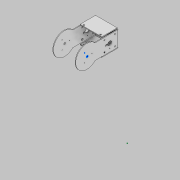
# Autodesk Inventor part: wzmocnienie2M1Dedit
Saved by Autodesk Inventor 2021 (Build 250183000, 183)
## iProperties
Created: 2021-09-03
Part Number: wzmocnienie2M1Dedit
Material: Ogólny
Document SubType Name: Konstrukcja blachowa
Designer: marci
Density: 1 g/cm^3
Sheet Metal Rule: Domyślny_mm
Appearance: Domyślna
Author: marci
Autodesk Inventor part; units mm, degrees
ref_plane "YZ Plane" through (0, 0, 0) normal (1, 0, 0) x (0, 1, 0)
sketch "Szkic1" plane through (0, 0, 0) normal (1, 0, 0) x (0, 1, 0)
  circle A0 centre (425.9063, 179.6758) radius 4.1
  line L0 (460.0949, 39.6758) -> (391.7177, 39.6758)
  line L1 (428.4063, 86.5216) -> (428.4063, 97.3591)
  line L2 (428.4063, 97.3591) -> (423.4063, 97.3591)
  line L3 (423.4063, 97.3591) -> (423.4063, 86.5216)
  arc A1 (423.4063, 86.5216) -> (428.4063, 86.5216) centre (425.9063, 77.8758) ccw
  circle A2 centre (406.1366, 78.0058) radius 1.65
  line L4 (460.0949, 143.191) -> (460.0949, 39.6758)
  arc A3 (460.0949, 143.191) -> (391.7177, 143.191) centre (425.9063, 179.6758) ccw
  line L5 (391.7177, 39.6758) -> (391.7177, 143.191)
  circle A4 centre (449.4563, 101.4258) radius 2.6
  circle A5 centre (402.3563, 101.4258) radius 2.6
  circle A6 centre (402.3563, 54.3258) radius 2.6
  circle A7 centre (449.4563, 54.3258) radius 2.6
  line L6 (423.4063, 95.8758) -> (428.4063, 95.8758)
  point P0 (0, 0)
  point P1 (391.7177, 143.191)
  dimension "d0" = 5.2
  dimension "d1" = 50
  dimension "d2" = 8.2
  dimension "d3" = 9
  dimension "d4" = 3.3
  dimension "d5" = 31.6886
  dimension "d6" = 36.6886
  dimension "d7" = 68.3772
  dimension "d8" = 1.4833
  dimension "d9" = 57.6833
  dimension "d10" = 0
  dimension "d11" = 45.8319
  dimension "d12" = 45.8319
  dimension "d13" = 57.6833
  dimension "d14" = 0
  dimension "d15" = 10.6386
  dimension "d16" = 4.0667
  dimension "d17" = 10.6386
  dimension "d18" = 43.0333
  dimension "d19" = 31.6886
  dimension "d20" = 0
  dimension "d21" = 31.6886
  dimension "d22" = 10.8375
  dimension "d23" = 31.6886
  dimension "d24" = 10.8375
  dimension "d25" = 34.1886
  dimension "d26" = 34.1886
  dimension "d27" = 36.6886
  dimension "d28" = 0
  dimension "d29" = 36.6886
  dimension "d30" = 10.8375
  dimension "d31" = 36.6886
  dimension "d32" = 22.2697
  dimension "d33" = 19.3533
  dimension "d34" = 57.7386
  dimension "d35" = 4.0667
  dimension "d36" = 57.7386
  dimension "d37" = 43.0333
  dimension "d38" = 68.3772
  dimension "d39" = 45.8319
  dimension "d40" = 68.3772
  dimension "d41" = 57.6833
  constraints: 14 end point, 8 centre point, 4 point on circle, 3 equal radius, 3 parallel, 3 perpendicular, 1 concentric
  measures "d0" diameter of A4
  measures "d1" radius of A3
  measures "d2" diameter of A0
  measures "d3" radius of A1
  measures "d4" diameter of A2
  measures "d5" distance between parallel lines of L4 L1
  measures "d6" distance between parallel lines of L4 L3
  measures "d7" distance between parallel lines of L4 L5
  measures "d8" distance between parallel lines of L6 L2
  measures "d9" distance between parallel lines of L2 L0
  measures "d10" distance from line of A3.start L4
  measures "d11" distance from line of A3.start L2
  measures "d12" distance from line of L4.start L2
  measures "d13" distance from line of L4.end L2
  measures "d14" distance from line of L0.start L4
  measures "d15" distance from line of A4.centre L4
  measures "d16" distance from line of A4.centre L2
  measures "d17" distance from line of A7.centre L4
  measures "d18" distance from line of A7.centre L2
  measures "d19" distance from line of L2.start L4
  measures "d20" distance from line of L1.end L2
  measures "d21" distance from line of L6.end L4
  measures "d22" distance from line of L1.start L2
  measures "d23" distance from line of A1.end L4
  measures "d24" distance from line of A1.end L2
  measures "d25" distance from line of A0.centre L4
  measures "d26" distance from line of A1.centre L4
  measures "d27" distance from line of L2.end L4
  measures "d28" distance from line of L3.start L2
  measures "d29" distance from line of L6.start L4
  measures "d30" distance from line of L3.end L2
  measures "d31" distance from line of A1.start L4
  measures "d32" distance from line of A2.centre L1
  measures "d33" distance from line of A2.centre L2
  measures "d34" distance from line of A5.centre L4
  measures "d35" distance from line of A5.centre L2
  measures "d36" distance from line of A6.centre L4
  measures "d37" distance from line of A6.centre L2
  measures "d38" distance from line of A3.end L4
  measures "d39" distance from line of L5.end L2
  measures "d40" distance from line of L0.end L4
  measures "d41" distance from line of L5.start L2
extrude "Wyciągnięcie proste1" add sketch "Szkic1" along normal blind 102.5
ref_plane "Płaszczyzna konstrukcyjna1" through (102.5, 425.9063, 229.6758) normal (0, 0, -1) x (-1, 0, 0)
sketch "Szkic2" plane through (102.5, 425.9063, 229.6758) normal (0, 0, -1) x (-1, 0, 0)
  line L0 (102.5, 50) -> (0, 50) projected
  line L1 (99.5, 50) -> (99.5, -50)
  line L2 (102.5, -50) -> (0, -50) projected
  line L3 (3, 50) -> (3, -50)
  line L4 (102.5, 50) -> (102.5, -50) projected
  line L5 (0, 50) -> (0, -50) projected
  line L6 (99.5, 50) -> (3, 50)
  line L7 (3, -50) -> (99.5, -50)
  point P0 (102.5, -425.9063)
  point P1 (102.5, 34.1886)
  point P2 (102.5, -34.1886)
  point P3 (0, 34.1886)
  point P4 (0, -34.1886)
  point P5 (3, 50)
  dimension "d44" = 3
  dimension "d45" = 3
  constraints: 8 end point, 2 point on line, 2 vertical, 1 collinear, 1 horizontal
  measures "d44" distance between parallel lines of L4 L1
  measures "d45" distance between parallel lines of L5 L3
extrude "Wyciągnięcie proste2" cut sketch "Szkic2" along normal blind 187 contours L1 L2 L3 L0
fillet "Zaokrąglenie1" radius 2 2 edges at (0, 425.9063, 39.6758) (102.5, 425.9063, 39.6758)
sketch "Szkic3" plane through (102.5, 0, 0) normal (1, 0, 0) x (0, 0, -1)
  circle A0 centre (-179.6758, 425.9063) radius 4.1 projected
  circle A1 centre (-179.6758, 425.9063) radius 50
  line L0 (-143.0152, 391.9063) -> (-39.6758, 391.9063)
  line L1 (-39.6758, 391.7177) -> (-39.6758, 460.0949) projected
  line L2 (-143.0152, 459.9063) -> (-39.6758, 459.9063)
  line L3 (-39.6758, 425.9063) -> (-57.2336, 425.9063)
  line L4 (-143.191, 391.7177) -> (-41.6758, 391.7177) projected
  line L5 (-41.6758, 460.0949) -> (-143.191, 460.0949) projected
  line L6 (-39.6758, 391.7177) -> (-41.6758, 391.7177) projected
  line L7 (-41.6758, 460.0949) -> (-39.6758, 460.0949) projected
  point P0 (0, 0)
  dimension "d49" = 68
  dimension "d50" = 34
  dimension "d51" = 100
  constraints: 6 end point, 2 horizontal, 2 point on circle, 2 point on line, 1 centre point, 1 coincident, 1 midpoint, 1 parallel
  measures "d49" distance between parallel lines of L2 L0
  measures "d50" distance between parallel lines of L3 L0
  measures "d51" diameter of A1
extrude "Wyciągnięcie proste3" cut sketch "Szkic3" against normal through all contours A1 L5 L7 L1 L2 | L0 L1 L6 L4 A1
sketch "Szkic4" plane through (102.5, 459.9063, 143.0152) normal (0, 1, 0) x (1, 0, 0)
  line L0 (-3, 100.3394) -> (-99.5, 100.3394) projected
  line L1 (-100.5, 103.3394) -> (-2, 103.3394) projected
  line L2 (-3, 100.3394) -> (-3, 103.3394)
  line L3 (-2, 103.3394) -> (-100.5, 103.3394) projected
  line L4 (0, 101.3394) -> (0, 0) projected
  line L5 (-99.5, 100.3394) -> (-99.5, 103.3394)
  point P0 (-102.5, 143.0152)
  point P1 (-3, 103.3394)
  dimension "d54" = 3
  constraints: 4 end point, 3 point on line, 2 perpendicular
  measures "d54" distance between parallel lines of L4 L2
extrude "Wyciągnięcie proste4" add sketch "Szkic4" along normal blind 3
ref_plane "Płaszczyzna konstrukcyjna2" through (102.5, 425.9063, 41.6758) normal (0, -1, 0) x (1, 0, 0)
mirror "Odbij1" about plane through (102.5, 425.9063, 41.6758) normal (0, -1, 0) of "Wyciągnięcie proste4"
sketch "Szkic5" plane through (2, 391.9063, 39.6758) normal (0, 0, -1) x (-1, 0, 0)
  line L0 (-1, 71) -> (-97.5, 71) projected
  line L1 (-97.5, 71) -> (-97.5, 74)
  line L2 (-97.5, -16) -> (-97.5, 84) projected
  line L3 (-97.5, 74) -> (-1, 74)
  line L4 (-1, -16) -> (-1, 84) projected
  line L5 (-1, 74) -> (-1, 71)
  line L6 (-1, 71) -> (-97.5, 71)
  line L7 (-97.5, 0) -> (-1, 0)
  line L8 (-1, 0) -> (-1, -3)
  line L9 (-1, -3) -> (-97.5, -3)
  line L10 (-97.5, -3) -> (-97.5, 0)
  point P0 (2, -391.9063)
  point P1 (-97.5, 68)
  point P2 (-1, 68)
  dimension "d57" = 3
  dimension "d58" = 3
  constraints: 16 end point, 3 parallel, 3 point on line, 2 perpendicular, 1 horizontal, 1 vertical
  measures "d57" distance of L0.end L1.end
  measures "d58" distance of L7.end L8.end
extrude "Wyciągnięcie proste5" add sketch "Szkic5" against normal blind 71 contours L0 L1 L3 L4
mirror "Odbij2" about plane through (102.5, 425.9063, 41.6758) normal (0, -1, 0) of "Wyciągnięcie proste5"
fillet "Zaokrąglenie2" radius 2 2 edges at (51.25, 465.9063, 39.6758) (51.25, 385.9063, 39.6758)
sketch "Szkic6" plane through (3, 385.9063, 110.6758) normal (0, -1, 0) x (1, 0, 0)
  circle A0 centre (85.5, -6) radius 2.85
  circle A1 centre (11, -6) radius 2.85
  line L0 (0, -69) -> (0, 0) projected
  line L1 (0, -71) -> (96.5, -71) projected
  line L2 (96.5, -69) -> (96.5, 0) projected
  point P0 (-3, -110.6758)
  dimension "d62" = 5.7
  dimension "d63" = 5.7
  dimension "d64" = 11
  dimension "d65" = 65
  dimension "d66" = 11
  dimension "d67" = 65
  constraints: 2 centre point
  measures "d62" diameter of A0
  measures "d63" diameter of A1
  measures "d64" distance from line of L0 A1.centre
  measures "d65" distance from line of L1 A1.centre
  measures "d66" distance from line of L2 A0.centre
  measures "d67" distance from line of L1 A0.centre
extrude "Wyciągnięcie proste6" cut sketch "Szkic6" against normal through all
sketch "Szkic7" plane through (99.5, 425.9063, 179.6758) normal (-1, 0, 0) x (0, 0, 1)
  circle A0 centre (-78.25, -23.55) radius 2.6 projected
  circle A1 centre (-78.25, -23.55) radius 6
  point P0 (-179.6758, -425.9063)
  dimension "d70" = 12
  constraints: 1 centre point, 1 coincident
  measures "d70" diameter of A1
chamfer "Faza1" distance 2 angle 45 1 edges at (99.5, 399.7563, 101.4258)
chamfer "Faza2" distance 2 angle 45 1 edges at (3, 399.7563, 101.4258)
sketch "Szkic8" plane through (102.5, 0, 0) normal (1, 0, 0) x (0, 0, -1)
  point P0 (-190.9258, 406.4207)
  point P1 (-190.9258, 445.3919)
  point P2 (-157.1758, 425.9063)
hole "Otwór1" at (102.5, 406.4207, 190.9258) at (102.5, 445.3919, 190.9258) at (102.5, 425.9063, 157.1758) direction (-1, 0, 0) diameter 2.459 depth 4.25 tip angle 120 thread size "M3x0.5" class "6H" standard "ISO Metric profile"
sketch "Szkic9" plane through (2, 391.9063, 39.6758) normal (0, 0, -1) x (-1, 0, 0)
  circle A0 centre (-49.25, 34) radius 4
  line L0 (-1, 74) -> (-97.5, 74) projected
  line L1 (-100.5, 68) -> (-100.5, 0) projected
  line L2 (-49.25, 34) -> (-93.3771, 34)
  line L3 (-49.25, 34) -> (-49.25, 64.9059)
  circle A1 centre (-87.25, 34) radius 3
  circle A2 centre (-49.25, 59) radius 3
  circle A3 centre (-11.25, 34) radius 3
  circle A4 centre (-49.25, 9) radius 3
  point P0 (2, -391.9063)
  dimension "d84" = 8
  dimension "d85" = 40
  dimension "d86" = 51.25
  dimension "d89" = 6
  dimension "d90" = 6
  dimension "d91" = 38
  dimension "d92" = 25
  dimension "d93" = 6
  dimension "d94" = 38
  dimension "d95" = 6
  dimension "d96" = 25
  constraints: 5 centre point, 4 end point, 2 point on line, 1 horizontal, 1 vertical
  measures "d84" diameter of A0
  measures "d85" distance from line of L0 L2.start
  measures "d86" distance from line of L1 L2.start
  measures "d89" diameter of A1
  measures "d90" diameter of A2
  measures "d91" distance of L2.start A1.centre
  measures "d92" distance of L2.start A2.centre
  measures "d93" diameter of A3
  measures "d94" distance of A3.centre L2.start
  measures "d95" diameter of A4
  measures "d96" distance of L2.start A4.centre
extrude "Wyciągnięcie proste7" cut sketch "Szkic9" against normal blind 71
sketch "Szkic10" plane through (0, 0, 0) normal (-1, 0, 0) x (0, 0, 1)
  point P0 (190.9258, 406.4207)
  point P1 (157.1758, 425.9063)
  point P2 (190.9258, 445.3919)
hole "Otwór2" at (0, 406.4207, 190.9258) at (0, 425.9063, 157.1758) at (0, 445.3919, 190.9258) direction (1, 0, 0) diameter 2.459 depth 4.25 tip angle 120 thread size "M3x0.5" class "6H" standard "ISO Metric profile"
sketch "Szkic11" plane through (102.5, 0, 0) normal (1, 0, 0) x (0, 0, -1)
  circle A0 centre (-190.9258, 445.3919) radius 1.2295 projected
  circle A1 centre (-190.9258, 445.3919) radius 1.2295
  circle A2 centre (-179.6758, 425.9063) radius 4.1 projected
  circle A3 centre (-179.6758, 425.9063) radius 4.1
  point P0 (0, 0)
  constraints: 2 centre point, 2 coincident
equation "\"PromieńGięcia\" = Grubość"
equation "\"SzerokośćGięciaPodcięcia\" = Grubość"
equation "\"GłębokośćGięciaPodcięcia\" = 0.5 * Grubość"
equation "\"RozmiarPodcięciaNarożnika\" = 4 * Grubość"
equation "\"MinimalnaPozostałość\" = 2 * Grubość"
equation "\"PromieńPrzejścia\" = PromieńGięcia"
equation "\"Rozmiar_promienia_Jacobiego\" = PromieńGięcia"
equation "\"Wielk_odstępu\" = Grubość"
equation "\"Grubość\" = 3"
